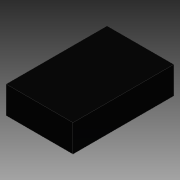
# Autodesk Inventor part: Fixture_Base_Support
Saved by Autodesk Inventor 2015 (Build 190159000, 159)
## iProperties
Created: 2014-12-16
Part Number: Fixture_Base_Support
Material: Generic
Document SubType Name: Modeling
Designer: amarschn
Density: 1 g/cm^3
Appearance: Anodized - Black
Author: amarschn
Autodesk Inventor part; units mm, degrees
ref_plane "YZ Plane" through (0, 0, 0) normal (1, 0, 0) x (0, 1, 0)
ref_plane "XZ Plane" through (0, 0, 0) normal (0, 1, 0) x (-1, 0, 0)
ref_plane "XY Plane" through (0, 0, 0) normal (0, 0, 1) x (1, 0, 0)
sketch "Sketch1" plane through (0, 0, 0) normal (0, 1, 0) x (-1, 0, 0)
  line L0 (-15.5575, -23.495) -> (15.5575, -23.495)
  line L1 (15.5575, -23.495) -> (15.5575, 23.495)
  line L2 (15.5575, 23.495) -> (-15.5575, 23.495)
  line L3 (-15.5575, 23.495) -> (-15.5575, -23.495)
  line L4 (-15.5575, -23.495) -> (15.5575, 23.495) construction
  line L5 (15.5575, -23.495) -> (-15.5575, 23.495) construction
  point P0 (0, 0)
  dimension "d0" = 46.99
  dimension "d1" = 31.115
  constraints: 12 end point, 2 midpoint, 2 parallel, 1 horizontal, 1 perpendicular
  measures "d0" distance of L0.end L1.end
  measures "d1" distance of L0.start L0.end
extrude "Extrusion1" add sketch "Sketch1" along normal blind 12.7
body "Solid1"
